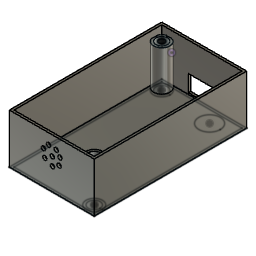
Assemblage TD01 groupe 04 (Autodesk Fusion 360 archive; units mm, degrees)
design "haut de la boite v6"
Autodesk Fusion 360 part; units mm, degrees
sketch "Sketch2" plane through (0, 0, 0) normal (0, 0, 1) x (1, 0, 0)
  line L0 (9.2902, -14.4648) -> (53.2902, -14.4648)
  line L1 (53.2902, -14.4648) -> (53.2902, -93.4648)
  line L2 (53.2902, -93.4648) -> (9.2902, -93.4648)
  line L3 (9.2902, -93.4648) -> (9.2902, -14.4648)
  line L4 (10.4902, -92.2648) -> (10.4902, -15.6648)
  line L5 (10.4902, -15.6648) -> (52.0902, -15.6648)
  line L6 (52.0902, -15.6648) -> (52.0902, -92.2648)
  line L7 (52.0902, -92.2648) -> (10.4902, -92.2648)
  circle A0 centre (14.2902, -19.4648) radius 4.2
  circle A1 centre (48.2902, -88.4648) radius 4.2
  circle A2 centre (14.2902, -19.4648) radius 3
  circle A3 centre (48.2902, -88.4648) radius 3
  circle A4 centre (41.5902, -21.9648) radius 5.5
  dimension "d5" = 44
  dimension "d6" = 79
  dimension "d9" = 14.4648
  dimension "d10" = 9.2902
  dimension "d11" = 1.2
  dimension "d16" = 8.4
  dimension "d19" = 8.4
  dimension "d55" = -1.2
  dimension "d56" = -1.2
  dimension "d61" = 11
  dimension "d66" = 6.3
  dimension "d67" = 10.5
  dimension "d116" = 3.8
  dimension "d117" = 3.8
  dimension "d118" = 3.8
  dimension "d119" = 3.8
  dimension "d120" = 6
  dimension "d121" = 6
  constraint horizontal L0
  constraint vertical L1
  constraint horizontal L2
  constraint vertical L3
  measures "d5" distance of L1 L3
  measures "d6" distance of L0 L2
  measures "d9" distance of origin L0
  measures "d10" distance of origin L3
  measures "d16" diameter of A0
  measures "d19" diameter of A1
  measures "d61" diameter of A4
  measures "d66" distance of L5 A4.centre
  measures "d67" distance of L6 A4.centre
  measures "d116" distance of L4 A0.centre
  measures "d117" distance of L5 A0.centre
  measures "d118" distance of L6 A1.centre
  measures "d119" distance of L7 A1.centre
  measures "d120" diameter of A2
  measures "d121" diameter of A3
extrude "Extrude15" add sketch "Sketch2" along normal blind 22 contours L4 A0 | L4 L5 A0 | L6 L7 A1 | L7 A1 | L6 A1 | L5 A0 picked at (14.2155, -15.9343) picked at (48.2155, -91.9954) makes body 1 at (18.4693, -19.0467, 14.6667) makes body 2 at (52.4693, -88.0467, 14.6667)
sketch "Sketch9" plane through (0, 0, 22) normal (0, 0, 1) x (-1, 0, 0)
  circle A0 centre (-14.2902, 19.4648) radius 3
  circle A1 centre (-14.2902, 19.4648) radius 4.2
  circle A2 centre (-14.2902, 19.4648) radius 1.5
  dimension "d177" = 3
  constraint concentric A0 A2
  measures "d177" diameter of A2
extrude "Extrude16" add sketch "Sketch2" along normal blind 1.2 contours L4 L5 L6 L7 A0 A1 bodies 1 2
extrude "Extrude17" add sketch "Sketch2" along normal blind 25.6 contours L0 L1 L2 L3 | L4 A0 | L7 A1 | L6 A1 | L5 A0 bodies 1
sketch "Sketch6" plane through (0, -14.4648, 0) normal (0, 1, 0) x (-1, 0, 0)
  line L0 (-53.2902, 0) -> (-9.2902, 0)
  line L1 (-9.2902, 0) -> (-9.2902, 25.6)
  line L2 (-9.2902, 25.6) -> (-53.2902, 25.6)
  line L3 (-53.2902, 25.6) -> (-53.2902, 0)
  line L4 (-38.2902, 2) -> (-24.2902, 2)
  line L5 (-24.2902, 2) -> (-24.2902, 10.6)
  line L6 (-24.2902, 10.6) -> (-38.2902, 10.6)
  line L7 (-38.2902, 10.6) -> (-38.2902, 2)
  line L8 (-9.2902, 0) -> (-53.2902, 0)
  dimension "d108" = 15
  dimension "d109" = 15
  dimension "d114" = 15
  dimension "d115" = 2
  constraint horizontal L4
  constraint vertical L5
  constraint horizontal L6
  constraint vertical L7
  measures "d108" distance of L3 L7
  measures "d109" distance of L1 L5
  measures "d114" distance of L2 L6
  measures "d115" distance of L4 L8
extrude "Extrude26" cut sketch "Sketch6" against normal blind 2 contours L4 L5 L6 L7 bodies 1
sketch "Sketch8" plane through (0, -93.4648, 0) normal (0, -1, 0) x (1, 0, 0)
  line L0 (9.2902, 0) -> (53.2902, 0)
  line L1 (53.2902, 0) -> (53.2902, 25.6)
  line L2 (53.2902, 25.6) -> (9.2902, 25.6)
  line L3 (9.2902, 25.6) -> (9.2902, 0)
  circle A0 centre (29.6137, 20.176) radius 1.1
  circle A1 centre (26.9669, 17.2485) radius 1.1
  circle A2 centre (27.6891, 13.3015) radius 1.1
  circle A3 centre (31.6361, 11.5132) radius 1.1
  circle A4 centre (35.0397, 13.5117) radius 1.1
  circle A5 centre (35.5472, 17.4587) radius 1.1
  circle A6 centre (33.5607, 19.8851) radius 1.1
  circle A7 centre (31.5499, 15.9058) radius 1.1
  dimension "d142" = 2.2
  dimension "d143" = 2.2
  dimension "d144" = 2.2
  dimension "d145" = 3.9467
  dimension "d146" = 3.947
  dimension "d150" = 2.2
  dimension "d151" = 2.2
  dimension "d153" = 3.947
  dimension "d155" = 3.947
  dimension "d156" = 2.2
  dimension "d159" = 3.947
  dimension "d160" = 2.2
  dimension "d162" = 3.947
  dimension "d163" = 17.743
  dimension "d164" = 8.1413
  dimension "d165" = 19.7295
  dimension "d166" = 5.7149
  dimension "d167" = 5.424
  dimension "d168" = 17.6767
  dimension "d169" = 18.2505
  dimension "d170" = 21.6541
  dimension "d171" = 2.2
  dimension "d172" = 21.7403
  dimension "d173" = 9.6942
  measures "d142" diameter of A0
  measures "d143" diameter of A1
  measures "d144" diameter of A2
  measures "d145" distance of A0.centre A1.centre
  measures "d146" vertical distance of A1.centre A2.centre
  measures "d150" diameter of A3
  measures "d151" diameter of A4
  measures "d153" horizontal distance of A2.centre A3.centre
  measures "d155" distance of A3.centre A4.centre
  measures "d156" diameter of A5
  measures "d159" vertical distance of A4.centre A5.centre
  measures "d160" diameter of A6
  measures "d162" horizontal distance of A0.centre A6.centre
  measures "d163" distance of L1 A5.centre
  measures "d164" distance of L2 A5.centre
  measures "d165" distance of L1 A6.centre
  measures "d166" distance of L2 A6.centre
  measures "d167" distance of L2 A0.centre
  measures "d168" distance of L3 A1.centre
  measures "d169" distance of L1 A4.centre
  measures "d170" distance of L1 A3.centre
  measures "d171" diameter of A7
  measures "d172" distance of L1 A7.centre
  measures "d173" distance of L2 A7.centre
hole "Hole5" at (33.5607, -93.4648, 19.8851) at (29.6137, -93.4648, 20.176) at (31.5499, -93.4648, 15.9058) at (26.9669, -93.4648, 17.2485) at (31.6361, -93.4648, 11.5132) at (27.6891, -93.4648, 13.3015) at (35.0397, -93.4648, 13.5117) at (35.5472, -93.4648, 17.4587) direction (0, 1, 0) diameter 2.2 depth 5 tip angle 118 bodies 1
sketch "Sketch7" plane through (0, 0, 0) normal (0, 0, -1) x (1, 0, 0)
  arc A0 (10.4902, 17.676) -> (12.5014, 15.6648) centre (14.2902, 19.4648) ccw
  line L0 (12.5014, 15.6648) -> (10.4902, 15.6648)
  line L1 (10.4902, 15.6648) -> (10.4902, 17.676)
  line L2 (53.2902, 93.4648) -> (9.2902, 93.4648)
  line L3 (9.2902, 93.4648) -> (9.2902, 14.4648)
  line L4 (9.2902, 14.4648) -> (53.2902, 14.4648)
  line L5 (53.2902, 14.4648) -> (53.2902, 93.4648)
  line L6 (50.0791, 92.2648) -> (52.0902, 92.2648)
  line L7 (52.0902, 92.2648) -> (52.0902, 90.2537)
  arc A1 (52.0902, 90.2537) -> (50.0791, 92.2648) centre (48.2902, 88.4648) ccw
  circle A2 centre (48.2902, 88.4648) radius 3
  circle A3 centre (41.5902, 21.9648) radius 5.5
  circle A4 centre (14.2902, 19.4648) radius 3
  line L8 (18.8193, 31.0267) -> (19.1397, 80.504) construction
  line L9 (19.1397, 80.504) -> (12.1251, 80.5494) construction
  line L10 (12.1251, 80.5494) -> (11.8048, 31.0721) construction
  line L11 (11.8048, 31.0721) -> (18.8193, 31.0267) construction
  dimension "d122" = 3
  text T0 "PEI TD1 Groupe 4" font "Arial" height 3 align centre top in box 49.4783 x 7.0147 at (18.8193, 31.0267) x (0.006474, 0.999979) y (-0.999979, 0.006474) spacing 1 kerned
extrude "Extrude27" add sketch "Sketch7" along normal blind 8 text T0 bodies 1
equation "d19 = d16"

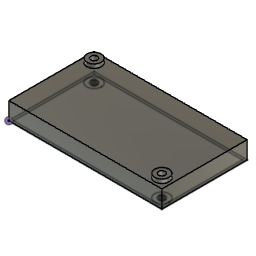
design "Bas Boite"
Autodesk Fusion 360 part; units mm, degrees
sketch "Sketch1" plane through (0, 0, 0) normal (0, 0, 1) x (1, 0, 0)
  line L0 (0, 0) -> (79, 0)
  line L1 (79, 0) -> (79, 44)
  line L2 (79, 44) -> (0, 44)
  line L3 (0, 44) -> (0, 0)
  circle A0 centre (5, 39) radius 1.7
  circle A1 centre (5, 39) radius 3.7
  circle A2 centre (74, 5) radius 1.7
  circle A3 centre (74, 5) radius 3.7
  line L4 (1.2, 42.8) -> (77.8, 42.8)
  line L5 (77.8, 42.8) -> (77.8, 1.2)
  line L6 (77.8, 1.2) -> (1.2, 1.2)
  line L7 (1.2, 1.2) -> (1.2, 42.8)
  dimension "d1" = 44
  dimension "d2" = 79
  dimension "d30" = 3.4
  dimension "d31" = 7.4
  dimension "d34" = 3.4
  dimension "d35" = 7.4
  dimension "d46" = 1.2
  dimension "d47" = 1.2
  dimension "d48" = 1.2
  dimension "d49" = 1.2
  dimension "d50" = 3.8
  dimension "d51" = 3.8
  dimension "d52" = 3.8
  dimension "d53" = 3.8
  constraint horizontal L0
  constraint vertical L1
  constraint horizontal L2
  constraint vertical L3
  constraint coincident L0.start L3.end
  constraint concentric A0 A1
  constraint concentric A2 A3
  constraint horizontal L4
  constraint vertical L5
  constraint horizontal L6
  constraint vertical L7
  measures "d1" distance of L0.start L2.end
  measures "d2" distance of L1.end L2.end
  measures "d30" diameter of A0
  measures "d31" diameter of A1
  measures "d34" diameter of A2
  measures "d35" diameter of A3
  measures "d46" distance of L3 L7
  measures "d47" distance of L2 L4
  measures "d48" distance of L0 L6
  measures "d49" distance of L1 L5
  measures "d50" distance of A2.centre L5
  measures "d51" distance of A2.centre L6
  measures "d52" distance of A0.centre L4
  measures "d53" distance of A0.centre L7
extrude "Extrude5" add sketch "Sketch1" along normal blind 11 contours A1 | A3 makes body 1 at (8.6954, 38.8156, 7.3333) makes body 2 at (77.6954, 4.8156, 7.3333)
extrude "Extrude6" add sketch "Sketch1" along normal blind 9 contours L0 L1 L2 L3 | L4 L5 L6 L7 bodies 1 2
extrude "Extrude7" cut sketch "Sketch1" along normal blind 2.6 contours A1 bodies 1
extrude "Extrude8" cut sketch "Sketch1" along normal blind 2.6 contours A0 | A1 | A3 bodies 1
